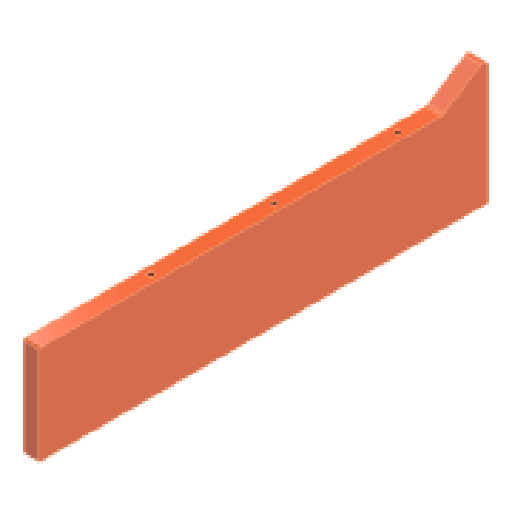
# Autodesk Inventor part: GRJ-04-102
Saved by Autodesk Inventor 2026.1 (Build 301233000, 233)
## iProperties
Company: Gree
Created: 2025-09-10
Part Number: GRJ-04-102
Material: Fenolite OR
Document SubType Name: Modeling
Designer: Willian Pinheiro
Density: 1.38 g/cm^3
Appearance: Suave - Laranja claro
Project: GRJ-04
Checked By: Antonio Lucas
Engr Approved By: Antonio Lucas
Description: Suporte Lateral
Mfg Approved By: Anderson Oliveira
Mass: 228.253 g
Surface Area: 409.938 cm^2
Volume: 165.401 cm^3
Dimensões: 10 x 80 x 273 mm
Total: 2
Author: Willian Pinheiro
Title: Pasta Dissipador G
Revision Number: 00
Autodesk Inventor part; units mm, degrees
ref_plane "YZ Plane" through (0, 0, 0) normal (1, 0, 0) x (0, 1, 0)
ref_plane "XZ Plane" through (0, 0, 0) normal (0, 1, 0) x (-1, 0, 0)
ref_plane "XY Plane" through (0, 0, 0) normal (0, 0, 1) x (1, 0, 0)
sketch "Sketch1" plane through (0, 0, 0) normal (1, 0, 0) x (0, 1, 0)
  line L0 (-191.1, 0) -> (191.1, 0) construction
  line L1 (0, -45.54) -> (0, 63.24) construction
  line L2 (-136.5, 30) -> (136.5, 30)
  line L3 (136.5, 30) -> (136.5, -30)
  line L4 (136.5, -30) -> (-136.5, -30)
  line L5 (-136.5, -30) -> (-136.5, 30)
  line L6 (109.0139, 30) -> (136.5, 47.7)
  line L7 (136.5, 47.7) -> (136.5, 30)
  circle A0 centre (133.5, 42.1999) radius 3
  circle A1 centre (115.5, 30.6086) radius 3
  line L8 (-136.5, 30) -> (103.5, 30) construction
  line L9 (103.5, 30) -> (103.5, 38) construction
  line L10 (103.5, 38) -> (-136.5, 38) construction
  line L11 (-136.5, 38) -> (-136.5, 30) construction
  line L12 (112.5, 32.2449) -> (112.5, 30)
  circle A2 centre (109.5, 30) radius 3
  circle A3 centre (109.5, 33) radius 3
  line L13 (-56.5, 30) -> (3.5, 30)
  line L14 (3.5, 30) -> (3.5, 6.4132)
  line L15 (3.5, 6.4132) -> (-56.5, 6.4132)
  line L16 (-56.5, 6.4132) -> (-56.5, 30)
  line L17 (-26.5, 6.4132) -> (-26.5, 30) construction
  point P0 (0, 0)
  point P1 (106.5, 30)
  dimension "d6" = 6
  dimension "d1" = 32.78
  dimension "d2" = 6
  dimension "d3" = 8
  dimension "d4" = 240
  dimension "d7" = 60
  dimension "d35" = 147.22
  dimension "d36" = 273
  dimension "d37" = 17.7
  dimension "d38" = 24
  dimension "d39" = 110
  dimension "d40" = 60
  constraints: 32 end point, 6 parallel, 6 tangent, 5 point on line, 3 centre point, 3 horizontal, 3 perpendicular, 2 midpoint, 2 vertical, 1 equal radius, 6 other
  measures "d1" angle of L2 L6
  measures "d2" diameter of A0
  measures "d3" distance between parallel lines of L2 L10
  measures "d4" distance of L9.end L10.end
  measures "d7" distance between parallel lines of L4 L2
  measures "d35" angle of L8 L6
  measures "d36" distance between parallel lines of L5 L7
  measures "d37" distance from line of L2 L6.end
  measures "d38" distance between parallel lines of L7 L12
  measures "d39" distance between parallel lines of L17 L5
  measures "d40" distance between parallel lines of L14 L16
extrude "Extrusion1" add sketch "Sketch1" along normal mid plane 10 contours L2 L16 L15 L14 A2 A1 L3 L4 L5 | L2 L14 L15 L16 | L2 A2 | L2 A1 L6 A0 L7 | L6 A3 L2 | L12 A1 L2 | A2 A3 L6 L12 | L2 A3 A2 | A1 L2 | L2 A1 | A0 L6 L7 | A0 | A3 L6 A2 | L6 A3 A2 | L12 L6 A1 picked at (110.4979, 30.6349) picked at (112.1863, 31.9825)
sketch "Sketch2" plane through (-5, -136.5, 30) normal (0, 0, 1) x (1, 0, 0)
  line L0 (5, -54.6) -> (5, 327.6) construction
  line L1 (0, 0) -> (10, 0) projected
  point P0 (5, 136.5)
  point P1 (5, 72.5)
  point P2 (5, 147.5)
  point P3 (5, 222.5)
  dimension "d11" = 72.5
  dimension "d12" = 75
  dimension "d13" = 75
  constraints: 3 point on line
  measures "d11" distance from line of point (5, 72.5) L1
  measures "d12" distance of point (5, 147.5) point (5, 72.5)
  measures "d13" distance of point (5, 222.5) point (5, 147.5)
hole "Hole1" at (0, -64, 30) at (0, 11, 30) at (0, 86, 30) direction (0, 0, -1) diameter 3.242 depth 15 tip angle 118 thread size "M4x0.7" class "6H" standard "ISO Metric profile"
sketch "Sketch3" plane through (5, 136.5, -30) normal (0, 0, -1) x (-1, 0, 0)
  line L0 (12, -136.5) -> (-2, -136.5) construction
  line L1 (5, -327.6) -> (5, 54.6) construction
  point P0 (5, -136.5)
  point P1 (5, -261.5)
  point P2 (5, -136.5)
  point P3 (5, -11.5)
  dimension "d21" = 250
  constraints: 1 coincident, 1 point on line, 1 symmetric about line
  measures "d21" distance of point (5, -11.5) point (5, -261.5)
hole "Hole2" at (0, -125, -30) at (0, 0, -30) at (0, 125, -30) direction (0, 0, 1) diameter 3.242 depth 15 tip angle 118 thread size "M4x0.7" class "6H" standard "ISO Metric profile"
fillet "Fillet1" radius 3 2 edges at (0, 136.5, 47.7) (0, 109.0139, 30)
chamfer "Chamfer1" distance 1 angle 45 1 edges at (0, -136.5, 30)
body "Solid1"
